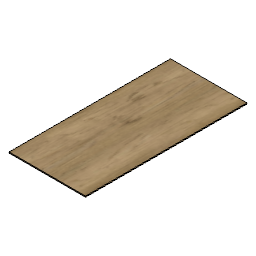
_Landing Shelf.48fbf440-f8d9-4674-903f-b4cdca804dc1 (Autodesk Fusion 360 design; units mm, degrees)
Autodesk Fusion 360 part; units mm, degrees
sketch "Sketch1" plane through (0, 0, 0) normal (0, 0, 1) x (1, 0, 0)
  line L0 (231.775, -488.95) -> (-231.775, -488.95)
  line L1 (-231.775, -488.95) -> (-231.775, 488.95)
  line L2 (-231.775, 488.95) -> (231.775, 488.95)
  line L3 (231.775, 488.95) -> (231.775, -488.95)
  line L4 (231.775, -488.95) -> (-231.775, 488.95) construction
  line L5 (-231.775, -488.95) -> (231.775, 488.95) construction
  dimension "d1" = 463.55
  dimension "d2" = 977.9
  constraint horizontal L0
  constraint perpendicular L0 L1
  constraint parallel L0 L2
  constraint parallel L1 L3
  constraint coincident L4 origin
  constraint coincident L5 origin
  measures "d1" distance of L1.end L2.end
  measures "d2" distance of L0.end L1.end
extrude "Extrude1" add sketch "Sketch1" along normal blind 6.35
